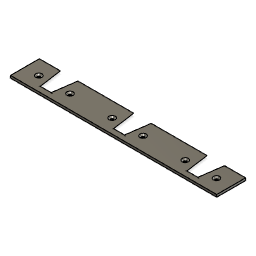
GNS530 Mount v2 v6 (Autodesk Fusion 360 archive; units mm, degrees)
design "CleatScratch"
Autodesk Fusion 360 part; units mm, degrees
sketch "Sketch1" plane through (0, 0, 0) normal (0, 1, 0) x (1, 0, 0)
  line L0 (0, 0) -> (0, 37)
  line L1 (0, 37) -> (22.3, 37)
  line L2 (22.3, 37) -> (26.5162, 7)
  line L3 (26.5162, 7) -> (50.5162, 7)
  line L4 (50.5162, 7) -> (54.7325, 37)
  line L5 (54.7325, 37) -> (115.85, 37)
  line L6 (115.85, 37) -> (120.0662, 7)
  line L7 (120.0662, 7) -> (132.0662, 7)
  line L8 (132.0662, 0) -> (0, 0)
  line L9 (38.5162, -8.148) -> (38.5162, 52.1011) construction
  line L10 (132.0662, 45.3898) -> (132.0662, -20) construction
  line L11 (38.5162, 16.5618) -> (132.0662, 16.5618) construction
  line L12 (85.2912, 3.5968) -> (85.2912, 70) construction
  line L13 (144.0662, 7) -> (132.0662, 7)
  line L14 (132.0662, 0) -> (264.1325, 0)
  line L15 (225.6162, 16.5618) -> (132.0662, 16.5618) construction
  line L16 (213.6162, 7) -> (209.4, 37)
  line L17 (264.1325, 0) -> (264.1325, 37)
  line L18 (209.4, 37) -> (148.2825, 37)
  line L19 (264.1325, 37) -> (241.8325, 37)
  line L20 (237.6162, 7) -> (213.6162, 7)
  line L21 (241.8325, 37) -> (237.6162, 7)
  line L22 (148.2825, 37) -> (144.0662, 7)
  circle A0 centre (245.8412, 18.0367) radius 1.95
  circle A1 centre (151.8412, 18) radius 1.95
  circle A2 centre (205.8412, 18) radius 1.95
  line L23 (151.8412, 18) -> (205.8412, 18) construction
  line L24 (178.8412, 30.7391) -> (178.8412, -7.4561) construction
  circle A3 centre (18.2912, 18.0367) radius 1.95
  circle A4 centre (58.2912, 18) radius 1.95
  circle A5 centre (112.2912, 18) radius 1.95
  line L25 (176, 66.8555) -> (176, -45) construction
  point P0 (85.2912, 16.5618)
  point P1 (38.5162, 7)
  point P2 (264.1325, 0)
  point P3 (132.0662, 45.3898)
  point P4 (225.6162, 7)
  point P5 (225.6162, -8.148)
  point P6 (178.8412, 3.5968)
  point P7 (178.8412, 16.5618)
  point P8 (-54791.8167, 16.4128)
  point P9 (178.8412, 18)
  dimension "d6" = 24
  dimension "d10" = 12
  dimension "d30" = 7
  dimension "d31" = 7
  dimension "d33" = 37
  dimension "d43" = 98
  dimension "d51" = 3.9
  dimension "d52" = 3.9
  dimension "d53" = 3.9
  dimension "d56" = 54
  dimension "d57" = 40
  dimension "d66" = 18
  dimension "d67" = 176
  constraint coincident L0.start L8.end
  constraint vertical L0
  constraint perpendicular L0 L1
  constraint perpendicular L8 L10
  constraint coincident L9 L11.start
  constraint coincident L10 L11.end
  constraint perpendicular L10 L11
  constraint perpendicular L11 L12
  constraint midpoint L11 P0
  constraint coincident L12 P0
  constraint coincident L7.end L10
  constraint midpoint L3 P1
  constraint coincident L9 P1
  constraint parallel L7 L8
  constraint parallel L5 L8
  constraint parallel L1 L8
  constraint collinear L1 L5
  constraint symmetric L2 L4 L9
  constraint parallel L2 L6
  constraint symmetric L0.start L10 P2
  constraint symmetric L0.end L10 L17.end
  constraint symmetric L1.end L10 L19.end
  constraint symmetric L2.end L10 L20.start
  constraint symmetric L3.end L10 L16.start
  constraint symmetric L4.end L10 L16.end
  constraint symmetric L5.end L10 L18.end
  constraint symmetric L6.end L10 L13.start
  constraint symmetric L7.end L10 L13.end
  constraint symmetric L8.start L10 L14.start
  constraint symmetric L9.start L10 P5
  constraint symmetric P3 L10 L10.start
  constraint symmetric L10 L11.start L15.start
  constraint symmetric L10 L11.end L15.end
  constraint symmetric L10 L12.start P6
  constraint symmetric L10 P0 P7
  constraint symmetric L10 P1 P4
  constraint coincident A1.centre L23.start
  constraint coincident A2.centre L23.end
  constraint parallel L15 L23
  constraint perpendicular L14 L24
  constraint midpoint L23 P9
  constraint coincident L24 P9
  constraint coincident P7 L24
  constraint symmetric L10 A0 A3
  constraint symmetric L10 A1 A5
  constraint symmetric L10 A2 A4
  constraint perpendicular L18 L25
  measures "d6" distance of L2.end L3.end
  measures "d10" distance of L6.end L7.end
  measures "d30" distance of L7.end L8.start
  measures "d31" distance of L3 L8
  measures "d33" distance of L0.start L0.end
  measures "d43" angle of L4 L5
  measures "d51" diameter of A0
  measures "d52" diameter of A1
  measures "d53" diameter of A2
  measures "d56" distance of A1.centre A2.centre
  measures "d57" distance of A0.centre A2.centre
  measures "d66" distance of L14 L23
  measures "d67" distance of L0 L25
ref_plane "WorkPlane1" through (0, -3, 0) normal (0, 1, 0) x (0, 0, 1)
sketch "Sketch3" plane through (0, -3, 0) normal (0, 1, 0) x (1, 0, 0)
  line L0 (127.4487, 7) -> (127.4487, 0)
  line L1 (116.2325, 37) -> (120.4487, 7)
  line L2 (44.7325, 37) -> (116.2325, 37)
  line L3 (21.5162, 7) -> (40.5162, 7)
  line L4 (-5, 37) -> (17.3, 37)
  line L5 (-5, 0) -> (-5, 37)
  line L6 (127.4487, 0) -> (-5, 0)
  line L7 (120.4487, 7) -> (127.4487, 7)
  line L8 (17.3, 37) -> (21.5162, 7)
  line L9 (116.2325, 37) -> (85.9376, 37) construction
  line L10 (40.5162, 7) -> (44.7325, 37)
  point P0 (-5, 0)
  dimension "d12" = 37
  dimension "d20" = 98
  dimension "d21" = 7
  dimension "d22" = 132.4487
  dimension "d23" = 19
  dimension "d26" = 98
  dimension "d27" = 98
  dimension "d28" = 7
  constraint coincident P0 L5.start
  constraint vertical L5
  constraint perpendicular L4 L5
  constraint horizontal L9
  constraint perpendicular L0 L6
  constraint parallel L3 L6
  constraint parallel L6 L7
  constraint parallel L2 L6
  constraint parallel L4 L6
  measures "d12" distance of P0 L4.start
  measures "d20" angle of L1 L9
  measures "d21" distance of L1.end L0.start
  measures "d22" distance of P0 L0.end
  measures "d23" distance of L3.end L3.start
  measures "d26" angle of L2 L10
  measures "d27" angle of L4 L8
  measures "d28" distance of L0.start L0.end
ref_plane "WorkPlane2" through (0, 3, 0) normal (0, 1, 0) x (0, 0, 1)
sketch "Sketch4" plane through (0, 3, 0) normal (0, 1, 0) x (1, 0, 0)
  line L0 (0, 37) -> (26.9487, 37)
  line L1 (143.2825, 37) -> (139.0662, 7)
  line L2 (264.1325, 0) -> (264.1325, 37)
  line L3 (38.1649, -7.8592) -> (38.1649, 52.3899) construction
  line L4 (232.9675, 7) -> (218.9675, 7)
  line L5 (214.7513, 37) -> (143.2825, 37)
  line L6 (38.1649, 16.8506) -> (132.0662, 16.8506) construction
  line L7 (225.9675, 16.8506) -> (132.0662, 16.8506) construction
  line L8 (31.1649, 7) -> (45.1649, 7)
  line L9 (218.9675, 7) -> (214.7513, 37)
  line L10 (237.1838, 37) -> (232.9675, 7)
  line L11 (139.0662, 7) -> (132.0662, 7)
  line L12 (26.9487, 37) -> (31.1649, 7)
  line L13 (132.0662, 45.6786) -> (132.0662, -19.7112) construction
  line L14 (264.1325, 37) -> (237.1838, 37)
  line L15 (85.1156, 3.8856) -> (85.1156, 70.2888) construction
  line L16 (49.3811, 37) -> (120.85, 37)
  line L17 (125.0662, 7) -> (132.0662, 7)
  line L18 (0, 0) -> (0, 37)
  line L19 (45.1649, 7) -> (49.3811, 37)
  line L20 (120.85, 37) -> (125.0662, 7)
  line L21 (0, 0) -> (264.1325, 0)
  point P0 (85.1156, 16.8506)
  point P1 (264.1325, 0)
  point P2 (225.9675, -7.8592)
  point P3 (132.0662, 45.6786)
  point P4 (225.9675, 7)
  point P5 (179.0169, 3.8856)
  point P6 (38.1649, 7)
  point P7 (179.0169, 16.8506)
  dimension "d45" = 14
  dimension "d46" = 7
  dimension "d49" = 37
  dimension "d50" = 98
  dimension "d54" = 7
  dimension "d55" = 7
  constraint coincident L18.start L21.start
  constraint vertical L18
  constraint perpendicular L0 L18
  constraint coincident L6.start L3
  constraint coincident L6.end L13
  constraint perpendicular L6 L13
  constraint perpendicular L6 L15
  constraint midpoint P0 L6
  constraint coincident P0 L15
  constraint coincident L11.end L13
  constraint midpoint P6 L8
  constraint coincident P6 L3
  constraint collinear L0 L16
  constraint symmetric L3 L12 L19
  constraint parallel L12 L20
  constraint symmetric P1 L18.start L13
  constraint symmetric L18.start P1 L13
  constraint symmetric L2.end L0.start L13
  constraint symmetric L0.end L10.start L13
  constraint symmetric L8.start L4.start L13
  constraint symmetric L8.end L4.end L13
  constraint symmetric L5.start L16.start L13
  constraint symmetric L1.start L16.end L13
  constraint symmetric L1.end L17.start L13
  constraint symmetric L11.end L17.end L13
  constraint symmetric P2 L3.start L13
  constraint symmetric P3 L13.start L13
  constraint symmetric L7.start L6.start L13
  constraint symmetric L6.end L7.end L13
  constraint symmetric P5 L15.start L13
  constraint symmetric P0 P7 L13
  constraint symmetric P4 P6 L13
  constraint collinear L4 L11
  measures "d45" distance of L8.end L8.start
  measures "d46" distance of L17.start L11.end
  measures "d49" distance of L18.start L0.start
  measures "d50" angle of L16 L19
  measures "d54" distance of L8 L21
  measures "d55" distance of L4 L21
loft "Loft1" add profiles "Sketch4", "Sketch1" section 1 section 2 contours L0 L1 L2 L3 L4 L5 L6 L7 L8 L13 L14 L16 L17 L18 L19 L20 L21 L22 | A0 | A1 | A2 | A3 | A4 | A5
extrude "Extrude1" cut sketch "Sketch1" along normal up to surface (3 mm away) contours A0 | A1 | A2 | A3 | A4 | A5
chamfer "Chamfer1" distance 2 angle 45 1 edges at (16.4732, 3, -18.7419)
chamfer "Chamfer2" distance 2 angle 45 1 edges at (56.4732, 3, -18.7052)
chamfer "Chamfer3" distance 2 angle 45 1 edges at (110.4732, 3, -18.7052)
chamfer "Chamfer4" distance 2 angle 45 1 edges at (150.0232, 3, -18.7052)
chamfer "Chamfer5" distance 2 angle 45 1 edges at (204.0232, 3, -18.7052)
chamfer "Chamfer6" distance 2 angle 45 1 edges at (244.0232, 3, -18.7419)
equation "d4 = 98 deg"
equation "d7 = d4"
equation "d10 = d6 / 2"
equation "d20 = d7"
equation "d26 = d20"
equation "d46 = d45 / 2"
